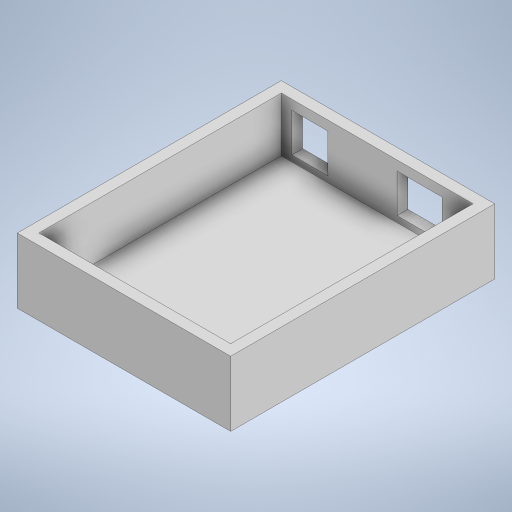
# Autodesk Inventor part: arduino array box v01
Saved by Autodesk Inventor 2023 (Build 270158000, 158)
## iProperties
Created: 2024-07-12
Part Number: arduino array box v01
Material: Generic
Document SubType Name: Modeling
Designer: Akramilab
Density: 1 g/cm^3
Appearance: Default
Author: Akramilab
Autodesk Inventor part; units mm, degrees
ref_plane "YZ Plane" through (0, 0, 0) normal (1, 0, 0) x (0, 1, 0)
ref_plane "XZ Plane" through (0, 0, 0) normal (0, 1, 0) x (-1, 0, 0)
ref_plane "XY Plane" through (0, 0, 0) normal (0, 0, 1) x (1, 0, 0)
sketch "Sketch2" plane through (0, 0, 0) normal (0, 1, 0) x (-1, 0, 0)
  line L0 (0, 0) -> (-59, 0)
  line L1 (-59, 0) -> (-59, 73)
  line L2 (-59, 73) -> (0, 73)
  line L3 (0, 73) -> (0, 0)
  dimension "d0" = 59
  dimension "d1" = 73
  constraints: 8 end point, 2 parallel, 1 horizontal, 1 perpendicular
  measures "d0" distance of L0.start L0.end
  measures "d1" distance between parallel lines of L2 L0
extrude "Extrusion1" add sketch "Sketch2" along normal blind 18
shell "Shell1" thickness 3 removed faces 1 at (19.6667, 18, 24.3333)
sketch "Sketch3" plane through (59, 0, 0) normal (0, 0, -1) x (-1, 0, 0)
  line L0 (11.5, 15.35) -> (24, 15.35)
  line L1 (24, 15.35) -> (24, 4.65)
  line L2 (24, 4.65) -> (11.5, 4.65)
  line L3 (11.5, 4.65) -> (11.5, 15.35)
  line L4 (0, 0) -> (0, 18) projected
  line L5 (0, 0) -> (59, 0) projected
  line L6 (43.1, 15.35) -> (53.1, 15.35)
  line L7 (53.1, 15.35) -> (53.1, 4.65)
  line L8 (53.1, 4.65) -> (43.1, 4.65)
  line L9 (43.1, 4.65) -> (43.1, 15.35)
  line L10 (59, 0) -> (59, 18) projected
  dimension "d5" = 11.5
  dimension "d6" = 4.65
  dimension "d7" = 12.5
  dimension "d8" = 10.7
  dimension "d10" = 10
  dimension "d11" = 10.7
  dimension "d12" = 4.65
  dimension "d16" = 43.1
  constraints: 16 end point, 4 parallel, 2 horizontal, 2 perpendicular
  measures "d5" distance between parallel lines of L4 L3
  measures "d6" distance between parallel lines of L5 L2
  measures "d7" distance of L0.start L0.end
  measures "d8" distance between parallel lines of L2 L0
  measures "d10" distance of L6.start L6.end
  measures "d11" distance of L8.end L6.start
  measures "d12" distance between parallel lines of L5 L8
  measures "d16" distance between parallel lines of L9 L4
extrude "Extrusion2" cut sketch "Sketch3" against normal blind 30
equation "\"d11\" = d8"
equation "\"d12\" = d6"
body "Solid1"
